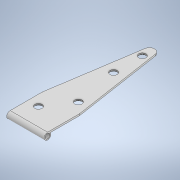
# Autodesk Inventor part: Ala 2 Bisagra tipo T
Saved by Autodesk Inventor 2020 (Build 240168000, 168)
## iProperties
Created: 2020-06-18
Part Number: Ala 2 Bisagra tipo T
Material: Genérico
Document SubType Name: Modeling
Designer: Pipi
Density: 1 g/cm^3
Appearance: Valor por defecto
Author: Pipi
Autodesk Inventor part; units mm, degrees
ref_plane "YZ Plane" through (0, 0, 0) normal (1, 0, 0) x (0, 1, 0)
ref_plane "XZ Plane" through (0, 0, 0) normal (0, 1, 0) x (-1, 0, 0)
ref_plane "XY Plane" through (0, 0, 0) normal (0, 0, 1) x (1, 0, 0)
sketch "Boceto1" plane through (0, 0, 0) normal (0, 1, 0) x (-1, 0, 0)
  line L0 (2.3676, 25.5961) -> (2.3676, 5.5961)
  line L1 (-23.6324, 5.5961) -> (-23.6324, 25.5961)
  line L2 (-23.6324, 25.5961) -> (2.3676, 25.5961)
  line L3 (2.3676, 25.5961) -> (2.3676, 5.5961)
  circle A0 centre (-16.1599, -0.9039) radius 2.5
  circle A1 centre (-4.9324, 15.5961) radius 2.5
  circle A2 centre (-10.6324, -50.9039) radius 2.5
  line L4 (2.3676, 5.5961) -> (-7.173, -56.436)
  line L5 (-14.0917, -56.436) -> (-23.6324, 5.5961)
  arc A3 (-14.0917, -56.436) -> (-7.173, -56.436) centre (-10.6324, -55.9039) ccw
  circle A4 centre (-10.6324, -30.9039) radius 2.5
  point P0 (0, 0)
  dimension "d2" = 20
  dimension "d16" = 26
  dimension "d17" = 5
  dimension "d18" = 5
  dimension "d19" = 5
  dimension "d20" = 10
  dimension "d21" = 7.3
  dimension "d22" = 26.5
  dimension "d26" = 5
  dimension "d30" = 5
  dimension "d31" = 20
  constraints: 12 end point, 5 centre point, 2 point on circle, 1 perpendicular, 1 tangent, 1 vertical
  measures "d2" distance of L0.end L0.start
  measures "d16" distance of L1.end L0.start
  measures "d17" diameter of A0
  measures "d18" diameter of A1
  measures "d19" diameter of A2
  measures "d20" distance from line of L2 A1.centre
  measures "d21" distance from line of L0 A1.centre
  measures "d22" distance from line of L2 A0.centre
  measures "d26" distance of A2.centre A3.centre
  measures "d30" diameter of A4
  measures "d31" distance of A4.centre A2.centre
extrude "Extrusión1" add sketch "Boceto1" along normal blind 1.2
sketch "Boceto4" plane through (23.6324, 0, 25.5961) normal (1, 0, 0) x (0, 0, -1)
  circle A0 centre (-2.375, -1.175) radius 2.375
  circle A1 centre (-2.375, -1.175) radius 1.625
  line L0 (0, 0) -> (0, 1.2) projected
  line L1 (0, 1.2) -> (20, 1.2) projected
  line L2 (20, 1.2) -> (0, 1.2) projected
  line L3 (0, 1.2) -> (-2.375, 1.2)
  line L4 (20, 0) -> (0, 0) projected
  line L5 (0, 0) -> (0, -1.175)
  point P0 (25.5961, 0)
  point P1 (20, 2)
  dimension "d12" = 4.75
  dimension "d13" = 3.25
  constraints: 4 end point, 2 centre point, 2 point on circle, 2 tangent, 1 coincident, 1 horizontal, 3 other
  measures "d12" diameter of A0
  measures "d13" diameter of A1
extrude "Extrusión3" add sketch "Boceto4" against normal blind 26
chamfer "Chaflán1" distance 0.25 angle 45 4 edges at (7.4324, 0, 15.5961) (18.6599, 0, -0.9039) (13.1324, 0, -50.9039) (13.1324, 0, -30.9039)
